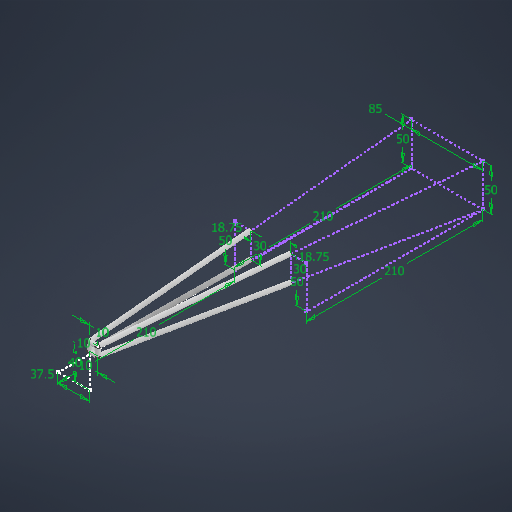
# Autodesk Inventor part: RCPlaneSkeletonTailRear1
Saved by Autodesk Inventor 2026.1 (Build 301233000, 233)
## iProperties
Created: 2026-03-11
Part Number: RCPlaneSkeletonTailRear1
Material: Generic
Document SubType Name: Modeling
Designer: morri
Density: 1 g/cm^3
Appearance: Default
Author: morri
Autodesk Inventor part; units mm, degrees
sketch3d "3D Sketch1"
ref_plane "Work Plane1" through (19.1234, 50.4741, -0.0556) normal (-0.0889319, 0, -0.9960377) x (0, -1, 0)
ref_plane "Work Plane2" through (66.6234, 50.4741, -0.0556) normal (0.0889319, 0, -0.9960377) x (0, 1, 0)
ref_plane "Work Plane3" through (19.1234, 20.4741, -0.0556) normal (-0.0885345, -0.0944368, -0.9915863) x (0.7295372, -0.6839411, 0)
ref_plane "Work Plane4" through (66.6234, 20.4741, -0.0556) normal (0.0885345, -0.0944368, -0.9915863) x (0.7295372, 0.6839411, 0)
sketch "Sketch1" plane through (19.1234, 50.4741, -0.0556) normal (-0.0889319, 0, -0.9960377) x (0, -1, 0)
  circle A0 centre (0, 0) radius 2.5
  point P0 (50.4741, 19.0525)
  dimension "d20" = 5
  constraints: 1 centre point
  measures "d20" diameter of A0
sketch "Sketch2" plane through (66.6234, 50.4741, -0.0556) normal (0.0889319, 0, -0.9960377) x (0, 1, 0)
  circle A0 centre (0, 0) radius 2.5
  point P0 (-50.4741, -66.3545)
  dimension "d21" = 5
  constraints: 1 centre point
  measures "d21" diameter of A0
sketch "Sketch3" plane through (19.1234, 20.4741, -0.0556) normal (-0.0885345, -0.0944368, -0.9915863) x (0.7295372, -0.6839411, 0)
  circle A0 centre (0, 0) radius 2.5
  point P0 (0.0519, 27.7874)
  dimension "d22" = 5
  constraints: 1 centre point
  measures "d22" diameter of A0
sketch "Sketch4" plane through (66.6234, 20.4741, -0.0556) normal (0.0885345, -0.0944368, -0.9915863) x (0.7295372, 0.6839411, 0)
  circle A0 centre (0, 0) radius 2.5
  point P0 (-62.6073, -30.3649)
  dimension "d23" = 5
  constraints: 1 centre point
  measures "d23" diameter of A0
sketch3d "3D Sketch2"
  line L0 (19.1234, 50.4741, -0.0556) -> (37.8734, 50.4741, 209.9444)
  dimension "d11" = 210
  dimension "d12" = 37.5
  dimension "d16" = 40
  dimension "d17" = 10
  dimension "d18" = 10
  dimension "d19" = 10
sweep "Sweep1" add profiles "Sketch1" path "3D Sketch2"
sketch3d "3D Sketch2 for Sweep2"
  line L0 (66.6234, 50.4741, -0.0556) -> (47.8734, 50.4741, 209.9444)
  dimension "d11" = 210
  dimension "d12" = 37.5
  dimension "d16" = 40
  dimension "d17" = 10
  dimension "d18" = 10
  dimension "d19" = 10
sweep "Sweep2" add profiles "Sketch2" path "3D Sketch2 for Sweep2" separate body
sketch3d "3D Sketch2 for Sweep3"
  line L0 (19.1234, 20.4741, -0.0556) -> (37.8734, 40.4741, 209.9444)
  dimension "d11" = 210
  dimension "d12" = 37.5
  dimension "d16" = 40
  dimension "d17" = 10
  dimension "d18" = 10
  dimension "d19" = 10
sweep "Sweep3" add profiles "Sketch3" path "3D Sketch2 for Sweep3" separate body
sketch3d "3D Sketch2 for Sweep4"
  line L0 (66.6234, 20.4741, -0.0556) -> (47.8734, 40.4741, 209.9444)
  dimension "d11" = 210
  dimension "d12" = 37.5
  dimension "d16" = 40
  dimension "d17" = 10
  dimension "d18" = 10
  dimension "d19" = 10
sweep "Sweep4" add profiles "Sketch4" path "3D Sketch2 for Sweep4" separate body
ref_plane "Work Plane5" through (37.8734, 50.4741, 209.9444) normal (-1, 0, 0) x (0, -1, 0)
ref_plane "Work Plane6" through (37.8734, 40.4741, 209.9444) normal (0, -1, 0) x (1, 0, 0)
sketch "Sketch6" plane through (37.8734, 50.4741, 209.9444) normal (-1, 0, 0) x (0, -1, 0)
  ellipse E0 centre (0, 0) end of major axis (2.5, 0) minor radius 0.2223 construction
  circle A0 centre (0, 0) radius 2.5
  ellipse E1 centre (10, 0) end of major axis (7.5113, -0.237) minor radius 0.2213 construction
  circle A1 centre (10, 0) radius 2.5
  point P0 (50.4741, -209.9444)
  dimension "d34" = 5
  dimension "d35" = 5
  constraints: 2 centre point, 2 coincident, 1 other
  measures "d34" diameter of A0
  measures "d35" diameter of A1
extrude "Extrusion1" add sketch "Sketch6" against normal blind 10 separate body
sketch "Sketch7" plane through (37.8734, 40.4741, 209.9444) normal (0, -1, 0) x (1, 0, 0)
  circle A0 centre (0, 0) radius 2.5
  line L0 (12.4901, 0.2223) -> (7.5099, -0.2223) construction
  circle A1 centre (10, 0) radius 2.5
  point P0 (-37.8734, -209.9444)
  dimension "d38" = 5
  dimension "d39" = 5
  constraints: 2 centre point, 1 midpoint
  measures "d38" diameter of A0
  measures "d39" diameter of A1
extrude "Extrusion2" add sketch "Sketch7" against normal blind 10 separate body
body "Solid1"
body "Solid2"
body "Solid3"
body "Solid4"
body "Solid5"
body "Solid6"
